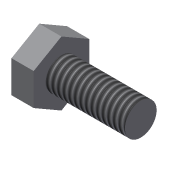
# Autodesk Inventor part: Šroub M3x8
Saved by Autodesk Inventor 2015 (Build 190159000, 159)
## iProperties
Created: 2015-01-09
Part Number: Šroub M3x8
Material: Všeobecné
Document SubType Name: Modeling
Designer: Michal
Density: 1 g/cm^3
Appearance: Výchozí
Author: Michal
Autodesk Inventor part; units mm, degrees
ref_plane "YZ Plane" through (0, 0, 0) normal (1, 0, 0) x (0, 1, 0)
ref_plane "XZ Plane" through (0, 0, 0) normal (0, 1, 0) x (-1, 0, 0)
ref_plane "XY Plane" through (0, 0, 0) normal (0, 0, 1) x (1, 0, 0)
sketch "Náčrt1" plane through (0, 0, 0) normal (1, 0, 0) x (0, 1, 0)
  line L0 (0, -4.0415) -> (-3.5, -2.0207)
  line L1 (-3.5, -2.0207) -> (-3.5, 2.0207)
  line L2 (-3.5, 2.0207) -> (0, 4.0415)
  line L3 (0, 4.0415) -> (3.5, 2.0207)
  line L4 (3.5, 2.0207) -> (3.5, -2.0207)
  line L5 (3.5, -2.0207) -> (0, -4.0415)
  point P0 (0, 0)
  point P1 (0, 0)
  dimension "d0" = 7
  constraints: 12 end point, 1 coincident, 13 other
  measures "d0" distance between parallel lines of L2 L5
extrude "Vysunutí1" add sketch "Náčrt1" along normal blind 2.8
sketch "Náčrt2" plane through (2.8, 0, 0) normal (1, 0, 0) x (0, 0, -1)
  circle A0 centre (0, 0) radius 2
  dimension "d3" = 4
  constraints: 1 centre point, 1 coincident
  measures "d3" diameter of A0
extrude "Vysunutí2" add sketch "Náčrt2" along normal blind 10
thread "Závit2" size "M4x0.7" class "6g" standard "ANSI Metric M Profile" full length
